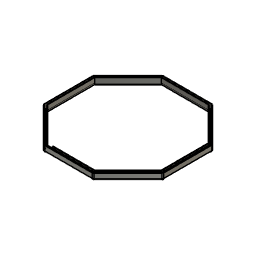
Projet_BAB3_Ring (Autodesk Fusion 360 design; units mm, degrees)
Autodesk Fusion 360 part; units mm, degrees
sketch "Esquisse1" plane through (0, 0, 0) normal (0, 0, 1) x (1, 0, 0)
  line L0 (-100, -41.4214) -> (-41.4214, -100)
  line L1 (-41.4214, -100) -> (41.4214, -100)
  line L2 (41.4214, -100) -> (100, -41.4214)
  line L3 (100, -41.4214) -> (100, 41.4214)
  line L4 (100, 41.4214) -> (41.4214, 100)
  line L5 (41.4214, 100) -> (-41.4214, 100)
  line L6 (-41.4214, 100) -> (-100, 41.4214)
  line L7 (-100, 41.4214) -> (-100, -41.4214)
  line L8 (-95, -39.3503) -> (-39.3503, -95)
  line L9 (-39.3503, -95) -> (39.3503, -95)
  line L10 (39.3503, -95) -> (95, -39.3503)
  line L11 (95, -39.3503) -> (95, 39.3503)
  line L12 (95, 39.3503) -> (39.3503, 95)
  line L13 (39.3503, 95) -> (-39.3503, 95)
  line L14 (-39.3503, 95) -> (-95, 39.3503)
  line L15 (-95, 39.3503) -> (-95, -39.3503)
extrude "Extrusion1" add sketch "Esquisse1" along normal blind 7 makes body 1
sketch "Esquisse2" plane through (0, 0, 7) normal (0, 0, 1) x (-1, 0, 0)
  line L0 (95, 39.3503) -> (95, -39.3503)
  line L1 (95, -39.3503) -> (39.3503, -95)
  line L2 (39.3503, -95) -> (-39.3503, -95)
  line L3 (-39.3503, -95) -> (-95, -39.3503)
  line L4 (-95, -39.3503) -> (-95, 39.3503)
  line L5 (-95, 39.3503) -> (-39.3503, 95)
  line L6 (-39.3503, 95) -> (39.3503, 95)
  line L7 (39.3503, 95) -> (95, 39.3503)
  line L8 (100, -41.4214) -> (100, 41.4214)
  line L9 (100, 41.4214) -> (41.4214, 100)
  line L10 (41.4214, 100) -> (-41.4214, 100)
  line L11 (-41.4214, 100) -> (-100, 41.4214)
  line L12 (-100, 41.4214) -> (-100, -41.4214)
  line L13 (-100, -41.4214) -> (-41.4214, -100)
  line L14 (-41.4214, -100) -> (41.4214, -100)
  line L15 (41.4214, -100) -> (100, -41.4214)
  line L16 (95, 0) -> (96, 0)
  line L17 (96, 0) -> (98.5, 0)
  line L18 (100, -41.4214) -> (95, -39.3503)
  line L19 (98.5, 0) -> (96, 0)
  line L20 (96, 0) -> (96, -40.8)
  line L21 (96, -40.8) -> (98.5, -40.8)
  line L22 (98.5, -40.8) -> (98.5, 0)
  line L23 (100, 41.4214) -> (95, 39.3503)
  line L24 (98.5, 0) -> (96, 0)
  line L25 (96, 0) -> (96, 40.8)
  line L26 (96, 40.8) -> (98.5, 40.8)
  line L27 (98.5, 40.8) -> (98.5, 0)
  dimension "d5" = 1
  dimension "d6" = 2.5
  constraint midpoint L0 L16.start
  constraint perpendicular L0 L16
  constraint perpendicular L0 L17
  constraint coincident L8.start L15.end
  constraint coincident L0.end L1.start
  constraint perpendicular L19 L20
  constraint parallel L19 L21
  constraint parallel L20 L22
  constraint coincident L8.end L9.start
  constraint coincident L0.start L7.end
  constraint perpendicular L24 L25
  constraint parallel L24 L26
  constraint parallel L25 L27
  measures "d5" distance of L16.start L16.end
  measures "d6" distance of L16.end L17.end
extrude "Extrusion2" cut sketch "Esquisse2" against normal blind 3 contours L17 L18 L19 L20 L22 L24 bodies 1
extrude "Extrusion3" cut sketch "Esquisse2" against normal blind 3 contours L17 L19 L23 L24 L25 L27 bodies 1
pattern_circular "Réseau C1" count 8 over 360 about axis through (0, 0, 1.75) along (0, 0, 1) of "Extrusion2", "Extrusion3"
ref_plane "Plan de construction2" through (-95, 0, 0) normal (-0.707107, 0, 0.707107) x (0, 1, 0)
sketch "Esquisse3" plane through (-47.5, 0, 47.5) normal (-0.707107, 0, 0.707107) x (0, 1, 0)
  line L0 (-40.7901, 68.425) -> (40.7901, 68.425)
  line L1 (40.7901, 68.425) -> (40.7901, 65.925)
  line L2 (40.7901, 65.925) -> (-40.7901, 65.925)
  line L3 (-40.7901, 65.925) -> (-40.7901, 68.425)
  line L4 (-40.7901, 68.425) -> (40.7901, 65.925) construction
  line L5 (40.7901, 68.425) -> (-40.7901, 65.925) construction
  point P0 (0, 67.175)
  dimension "d15" = 2.5
  constraint horizontal L0
  constraint perpendicular L0 L1
  constraint parallel L0 L2
  constraint parallel L1 L3
  constraint coincident L4 P0
  constraint coincident L5 P0
  measures "d15" distance of L0.end L1.end
extrude "Extrusion4" cut sketch "Esquisse3" along normal blind 4 bodies 1
extrude "Extrusion5" cut sketch "Esquisse3" against normal blind 3 bodies 1
pattern_circular "Réseau C2" count 8 over 360 about axis through (0, 0, 1.75) along (0, 0, 1) of "Extrusion4", "Extrusion5"
fillet "Congé1" radius 3 8 edges at (-100, 0, 0) (-70.7107, 70.7107, 0) (0, 100, 0) (70.7107, 70.7107, 0) (100, 0, 0) (70.7107, -70.7107, 0) (0, -100, 0) (-70.7107, -70.7107, 0) on bodies 1
extrude "Extrusion8" add 1 faces at (60.7405, -79.9738, 7) along direction (0, 0, 1) blind 5 on bodies 1 bodies 1
sketch "Esquisse4" plane through (0, 0, 7) normal (0, 0, 1) x (-1, 0, 0)
  line L0 (39.7645, -96) -> (96, -39.7645)
  line L1 (96, -39.7645) -> (96, 39.7645)
  line L2 (96, 39.7645) -> (39.7645, 96)
  line L3 (39.7645, 96) -> (-39.7645, 96)
  line L4 (-39.7645, 96) -> (-96, 39.7645)
  line L5 (-96, 39.7645) -> (-96, -39.7645)
  line L6 (-96, -39.7645) -> (-39.7645, -96)
  line L7 (-39.7645, -96) -> (39.7645, -96)
  line L8 (95, 39.3503) -> (95, -39.3503)
  line L9 (95, -39.3503) -> (39.3503, -95)
  line L10 (39.3503, -95) -> (-39.3503, -95)
  line L11 (-39.3503, -95) -> (-95, -39.3503)
  line L12 (-95, -39.3503) -> (-95, 39.3503)
  line L13 (-95, 39.3503) -> (-39.3503, 95)
  line L14 (-39.3503, 95) -> (39.3503, 95)
  line L15 (39.3503, 95) -> (95, 39.3503)
  line L16 (39.7645, 96) -> (30.4715, 96)
  line L17 (39.7645, 96) -> (46.3356, 89.4289)
  line L18 (30.4715, 96) -> (37.0426, 89.4289)
  line L19 (37.0426, 89.4289) -> (46.3356, 89.4289)
  dimension "d42" = 9.293
  dimension "d43" = 9.293
  dimension "d44" = 9.293
  constraint coincident L2.end L3.start
  constraint coincident L3 L16.end
  constraint parallel L2 L17
  constraint parallel L17 L18
  measures "d42" distance of L2.end L16.end
  measures "d43" distance of L2.end L17.end
  measures "d44" distance of L16.end L18.end
extrude "Extrusion6" cut sketch "Esquisse4" against normal blind 6 contours L2 L3 L14 L15 L16 L17 L18 L19 bodies 1
sketch "Esquisse5" plane through (0, 0, 4) normal (0, 0, 1) x (-1, 0, 0)
  line L0 (98.5, -40.8) -> (98.5, 40.8)
  line L1 (98.5, 40.8) -> (40.8, 98.5)
  line L2 (40.8, 98.5) -> (-40.8, 98.5)
  line L3 (-40.8, 98.5) -> (-98.5, 40.8)
  line L4 (-98.5, 40.8) -> (-98.5, -40.8)
  line L5 (-98.5, -40.8) -> (-40.8, -98.5)
  line L6 (-40.8, -98.5) -> (40.8, -98.5)
  line L7 (40.8, -98.5) -> (98.5, -40.8)
  line L8 (96, -39.7645) -> (39.7645, -96)
  line L9 (39.7645, -96) -> (-39.7645, -96)
  line L10 (-39.7645, -96) -> (-96, -39.7645)
  line L11 (-96, -39.7645) -> (-96, 39.7645)
  line L12 (-96, 39.7645) -> (-39.7645, 96)
  line L13 (-39.7645, 96) -> (30.4715, 96)
  line L14 (30.4715, 96) -> (39.7645, 96)
  line L15 (39.7645, 96) -> (46.3356, 89.4289)
  line L16 (46.3356, 89.4289) -> (96, 39.7645)
  line L17 (96, 39.7645) -> (96, -39.7645)
  line L18 (40.8, 98.5) -> (39.7645, 96)
  line L19 (40.8, 98.5) -> (35.118, 84.7824)
  line L20 (40.8, 98.5) -> (33.7199, 81.407)
  line L21 (30.4715, 96) -> (34.818, 84.0581)
  line L22 (30.4715, 96) -> (43.1798, 96) construction
  line L23 (46.3356, 89.4289) -> (34.818, 84.0581)
  dimension "d47" = 70
  constraint coincident L1.end L2.start
  constraint coincident L14.end L15.start
  constraint parallel L18 L19
  constraint parallel L18 L20
  constraint horizontal L22
  constraint coincident L13.end L14.start
  constraint coincident L20 L21.end
  constraint coincident L15.end L16.start
  measures "d47" angle of L21 L22
extrude "Extrusion7" cut sketch "Esquisse5" along normal mid plane 12 contours L15 L19 L20 L23 | L14 L19 L20 L21 bodies 1
copy_body "Corps->Comp1" bodies 1 removing the originals makes body 2 in component "Component"
sketch "Esquisse6" plane through (0, 0, 7) normal (0, 0, 1) x (-1, 0, 0)
  line L0 (30.8355, 95) -> (30.4715, 96)
  line L1 (30.4715, 96) -> (-39.7645, 96)
  line L2 (-39.7645, 96) -> (-96, 39.7645)
  line L3 (-96, 39.7645) -> (-96, -39.7645)
  line L4 (-96, -39.7645) -> (-39.7645, -96)
  line L5 (-39.7645, -96) -> (39.7645, -96)
  line L6 (39.7645, -96) -> (96, -39.7645)
  line L7 (96, -39.7645) -> (96, 39.7645)
  line L8 (96, 39.7645) -> (46.3356, 89.4289)
  line L9 (46.3356, 89.4289) -> (45.3712, 88.9791)
  line L10 (45.3712, 88.9791) -> (95, 39.3503)
  line L11 (95, 39.3503) -> (95, -39.3503)
  line L12 (95, -39.3503) -> (39.3503, -95)
  line L13 (39.3503, -95) -> (-39.3503, -95)
  line L14 (-39.3503, -95) -> (-95, -39.3503)
  line L15 (-95, -39.3503) -> (-95, 39.3503)
  line L16 (-95, 39.3503) -> (-39.3503, 95)
  line L17 (-39.3503, 95) -> (30.8355, 95)
extrude "Extrusion1'" add sketch "Esquisse6" along normal blind 5 bodies 2 in component "Component"
fillet "Congé1'" radius 1 8 edges at (-70.7107, 70.7107, 12) (0, 100, 12) (70.7107, 70.7107, 12) (100, 0, 12) (70.7107, -70.7107, 12) (0, -100, 12) (-70.7107, -70.7107, 12) (-100, 0, 12) on bodies 2 in component "Component"
fillet "Congé2" radius 3 24 edges at (99.1213, 41.0574, 0.8787) (100, 41.4214, 7) (99.7071, 41.3, 11.7071) (99.1213, -41.0574, 0.8787) (100, -41.4214, 7) (99.7071, -41.3, 11.7071) (41.0574, 99.1213, 0.8787) (41.4214, 100, 7) (41.3, 99.7071, 11.7071) (-41.0574, 99.1213, 0.8787) (-41.4214, 100, 7) (-41.3, 99.7071, 11.7071) (-99.1213, 41.0574, 0.8787) (-100, 41.4214, 7) (-99.7071, 41.3, 11.7071) (-99.1213, -41.0574, 0.8787) (-100, -41.4214, 7) (-99.7071, -41.3, 11.7071) (-41.0574, -99.1213, 0.8787) (-41.4214, -100, 7) (-41.3, -99.7071, 11.7071) (41.0574, -99.1213, 0.8787) (41.4214, -100, 7) (41.3, -99.7071, 11.7071) on bodies 2 in component "Component"
ref_plane "Plan de construction4" through (-40.1787, -100, 3) normal (0.382683, 0.92388, 0) x (-0.92388, 0.382683, 0)
sketch "Esquisse8" plane through (-41.2394, -99.5607, 0) normal (0.382683, 0.92388, 0) x (-0.92388, 0.382683, 0)
  circle A0 centre (0, 7) radius 3
  dimension "d61" = 6
  measures "d61" diameter of A0
extrude "Extrusion3'" cut sketch "Esquisse8" along normal mid plane 18 bodies 2 in component "Component"
component "Component" placed x (1, 0, 0) y (0, 1, 0) z (0, 0, 1) at (0, 0, 0)
